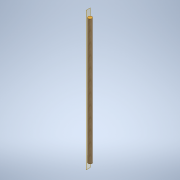
# Autodesk Inventor part: leadscrew
Saved by Autodesk Inventor 2020 (Build 240168000, 168)
## iProperties
Created: 2020-12-23
Part Number: leadscrew
Material: Generic
Document SubType Name: Modeling
Designer: Vikki
Density: 1 g/cm^3
Appearance: Brass - Satin
Author: Vikki
Autodesk Inventor part; units mm, degrees
ref_plane "XZ Plane" through (0, 0, 0) normal (0, 1, 0) x (-1, 0, 0)
ref_plane "XY Plane" through (0, 0, 0) normal (0, 0, 1) x (1, 0, 0)
sketch "Sketch1" plane through (0, 0, 0) normal (0, 1, 0) x (-1, 0, 0)
  circle A0 centre (0, 0) radius 3
  dimension "d0" = 6
  constraints: 1 centre point, 1 coincident
  measures "d0" diameter of A0
extrude "Extrusion1" add sketch "Sketch1" along normal blind 200
thread "Thread1" size "TR8x1.5" class "7e" standard "ISO Metric Trapezoidal Threads" full length
ref_plane "Work Plane1" through (-3, 0, 0) normal (1, 0, 0) x (0, 1, 0)
sketch "Sketch2" plane through (-3, 0, 0) normal (1, 0, 0) x (0, 1, 0)
  line L0 (0, -5) -> (0, 5)
  line L1 (0, 5) -> (10, 5)
  line L2 (10, 5) -> (10, -5)
  line L3 (10, -5) -> (0, -5)
  line L4 (0, 3) -> (200, 3) projected
  point P0 (0, 0)
  point P1 (10, 3)
  dimension "d5" = 10
  dimension "d6" = 10
  dimension "d7" = 5
  constraints: 8 end point, 2 parallel, 2 perpendicular, 1 midpoint
  measures "d5" distance of L0.start L0.end
  measures "d6" distance of L0.end L1.end
  measures "d7" distance of L0.end point (0, 0)
extrude "Extrusion2" cut sketch "Sketch2" along normal blind 1.5 contours L0 L4 L2 L3
equation "\"d7\" = 0.5 * d5"
body "Solid1"
